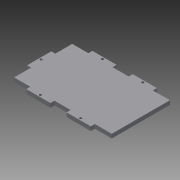
# Autodesk Inventor part: top
Saved by Autodesk Inventor 2014 (Build 180170000, 170)
## iProperties
Created: 2014-03-02
Part Number: top
Material: 常规
Document SubType Name: Modeling
Designer: Keshuai
Density: 1 g/cm^3
Appearance: 默认
Author: Keshuai
Autodesk Inventor part; units mm, degrees
ref_plane "YZ Plane" through (0, 0, 0) normal (1, 0, 0) x (0, 1, 0)
ref_plane "XZ Plane" through (0, 0, 0) normal (0, 1, 0) x (-1, 0, 0)
ref_plane "XY Plane" through (0, 0, 0) normal (0, 0, 1) x (1, 0, 0)
sketch "草图1" plane through (0, 0, 0) normal (0, 0, 1) x (1, 0, 0)
  line L0 (0, -72) -> (0, 0) projected
  line L1 (0, 0) -> (116, 0) projected
  line L2 (116, 0) -> (116, -72) projected
  line L3 (121, 0) -> (121, -72) projected
  line L4 (121, 0) -> (0, 0)
  line L5 (0, 0) -> (0, -72)
  line L6 (0, -72) -> (121, -72)
  line L7 (121, -72) -> (121, 0)
  line L8 (20, 0) -> (50, 0)
  line L9 (50, 0) -> (50, 5)
  line L10 (50, 5) -> (20, 5)
  line L11 (20, 5) -> (20, 0)
  line L12 (70, 0) -> (100, 0)
  line L13 (100, 0) -> (100, 5)
  line L14 (100, 5) -> (70, 5)
  line L15 (70, 5) -> (70, 0)
  line L16 (-14.7833, -36) -> (35, -36) construction
  line L17 (-5, -21) -> (0, -21)
  line L18 (0, -21) -> (0, -51)
  line L19 (0, -51) -> (-5, -51)
  line L20 (-5, -51) -> (-5, -21)
  line L21 (20, -72) -> (50, -72)
  line L22 (50, -72) -> (50, -77)
  line L23 (50, -77) -> (20, -77)
  line L24 (20, -77) -> (20, -72)
  line L25 (70, -72) -> (100, -72)
  line L26 (100, -72) -> (100, -77)
  line L27 (100, -77) -> (70, -77)
  line L28 (70, -77) -> (70, -72)
  circle A0 centre (35, 2.5) radius 1.5
  circle A1 centre (85, 2.5) radius 1.5
  circle A2 centre (-2.5, -36) radius 1.5
  circle A3 centre (35, -74.5) radius 1.5
  circle A4 centre (85, -74.5) radius 1.5
  point P0 (-5, -72)
  point P1 (-5, 0)
  point P2 (0, 5)
  point P3 (116, 5)
  point P4 (0, -36)
  dimension "d0" = 30
  dimension "d1" = 30
  dimension "d2" = 20
  dimension "d3" = 20
  dimension "d4" = 5
  dimension "d5" = 30
  dimension "d6" = 5
  dimension "d7" = 3
  dimension "d8" = 3
  dimension "d9" = 3
  dimension "d10" = 3
  dimension "d11" = 3
  constraints: 50 end point, 12 parallel, 7 horizontal, 7 perpendicular, 6 point on line, 5 centre point, 1 collinear, 1 midpoint, 4 other
  measures "d0" distance of L10.end L9.end
  measures "d1" distance of L14.end L13.end
  measures "d2" distance between parallel lines of L5 L11
  measures "d3" distance between parallel lines of L15 L9
  measures "d4" distance of L18.end L19.end
  measures "d5" distance of L17.end L18.end
  measures "d6" distance of L21.end L22.end
  measures "d7" diameter of A0
  measures "d8" diameter of A1
  measures "d9" diameter of A2
  measures "d10" diameter of A3
  measures "d11" diameter of A4
extrude "拉伸1" add sketch "草图1" along normal blind 5
